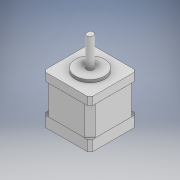
# Autodesk Inventor part: NEMA_14_Dual_LM1048
Saved by Autodesk Inventor 2020.3 (Build 243373000, 373)
## iProperties
Created: 2020-05-16
Part Number: NEMA_14_Dual_LM1048
Material: Generic
Document SubType Name: Modeling
Designer: rah75
Density: 1 g/cm^3
Appearance: Default
Author: rah75
Autodesk Inventor part; units mm, degrees
ref_plane "YZ Plane" through (0, 0, 0) normal (1, 0, 0) x (0, 1, 0)
sketch "Sketch1" plane through (0, 0, 0) normal (0, 1, 0) x (-1, 0, 0)
  line L0 (-17.6, 17.6) -> (17.6, 17.6)
  line L1 (17.6, 17.6) -> (17.6, -17.6)
  line L2 (17.6, -17.6) -> (-17.6, -17.6)
  line L3 (-17.6, -17.6) -> (-17.6, 17.6)
  line L4 (-17.6, 17.6) -> (17.6, -17.6) construction
  line L5 (17.6, 17.6) -> (-17.6, -17.6) construction
  point P0 (0, 0)
  dimension "d0" = 35.2
  dimension "d1" = 35.2
  constraints: 12 end point, 2 midpoint, 2 parallel, 1 horizontal, 1 perpendicular
  measures "d0" distance of L1.end L2.end
  measures "d1" distance of L0.end L1.end
extrude "Extrusion1" add sketch "Sketch1" along normal mid plane 36
sketch "Sketch2" plane through (0, 18, 0) normal (0, 1, 0) x (1, 0, 0)
  circle A0 centre (0, 0) radius 11
  dimension "d4" = 22
  constraints: 1 centre point, 1 coincident
  measures "d4" diameter of A0
extrude "Extrusion2" add sketch "Sketch2" along normal blind 2
sketch "Sketch3" plane through (0, 18, 0) normal (0, 1, 0) x (1, 0, 0)
  circle A0 centre (0, 0) radius 2.5
  dimension "d7" = 5
  constraints: 1 centre point, 1 coincident
  measures "d7" diameter of A0
extrude "Extrusion3" add sketch "Sketch3" along normal blind 24
sketch "Sketch4" plane through (0, 42, 0) normal (0, 1, 0) x (1, 0, 0)
  circle A0 centre (0, 0) radius 2.5 projected
  line L0 (-2, -1.5) -> (-2, 1.5)
  circle A1 centre (0, 0) radius 2.5 projected
  dimension "d10" = 4.5
  constraints: 2 end point, 2 point on circle, 1 vertical
extrude "Extrusion4" cut sketch "Sketch4" against normal blind 15 contours L0 A0 picked at (-2.0912, -0.3466)
ref_plane "Work Plane2" through (0, 12, 0) normal (0, 1, 0) x (1, 0, 0)
ref_plane "Work Plane1" through (0, -10, 0) normal (0, -1, 0) x (1, 0, 0)
sketch "Sketch5" plane through (0, -10, 0) normal (0, -1, 0) x (1, 0, 0)
  line L0 (-17.6, -17.6) -> (17.6, -17.6) projected
  line L1 (17.6, -17.6) -> (17.6, 17.6) projected
  line L2 (17.6, 17.6) -> (-17.6, 17.6) projected
  line L3 (-17.6, 17.6) -> (-17.6, -17.6) projected
  line L4 (-17.59, -17.59) -> (17.59, -17.59)
  line L5 (17.59, -17.59) -> (17.59, 17.59)
  line L6 (17.59, 17.59) -> (-17.59, 17.59)
  line L7 (-17.59, 17.59) -> (-17.59, -17.59)
  point P0 (0, 0)
  dimension "d14" = 0.01
  constraints: 8 end point, 3 other
  measures "d14" distance between parallel lines of L3 L7
extrude "Extrusion5" cut sketch "Sketch5" against normal up to surface (22 mm away)
chamfer "Chamfer1" distance 4 angle 45 4 edges at (-17.59, 1, 17.59) (-17.59, 1, -17.59) (17.59, 1, 17.59) (17.59, 1, -17.59)
chamfer "Chamfer2" distance 2 angle 45 8 edges at (-17.6, 15, 17.6) (-17.6, -14, 17.6) (17.6, 15, 17.6) (17.6, -14, 17.6) (-17.6, -14, -17.6) (17.6, 15, -17.6) (17.6, -14, -17.6) (-17.6, 15, -17.6)
sketch "Sketch6" plane through (0, -18, 0) normal (0, -1, 0) x (1, 0, 0)
  circle A0 centre (0, 0) radius 2.5 projected
  circle A1 centre (0, 0) radius 2.5
  dimension "d24" = 5
  constraints: 1 centre point, 1 coincident
  measures "d24" diameter of A1
extrude "Extrusion6" add sketch "Sketch6" along normal blind 13
fillet "Fillet1" radius 1 1 edges at (-2.5, -31, 0)
sketch "Sketch7" plane through (0, -18, 0) normal (0, -1, 0) x (1, 0, 0)
  circle A0 centre (0, 0) radius 1.5 projected
  circle A1 centre (0, 0) radius 9.525
  point P0 (-9.525, 0)
  point P1 (9.525, 0)
  dimension "d28" = 19.05
  constraints: 2 horizontal alignment, 2 point on circle, 1 centre point, 1 coincident
  measures "d28" diameter of A1
hole "Hole1" at (-9.525, -18, 0) at (9.525, -18, 0) direction (0, 1, 0) diameter 2.013 depth 7.6 tip angle 118 thread size "M2.5x0.45" class "6H" standard "ANSI Metric M Profile"
body "Solid1"
